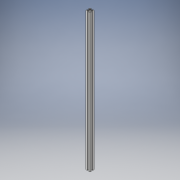
# Autodesk Inventor part: pro36in
Saved by Autodesk Inventor 2018 (Build 220112000, 112)
## iProperties
Created: 2017-09-02
Part Number: pro36in
Material: Generic
Document SubType Name: Modeling
Designer: snipe
Density: 1 g/cm^3
Appearance: Default
Author: snipe
Autodesk Inventor part; units mm, degrees
ref_plane "YZ Plane" through (0, 0, 0) normal (1, 0, 0) x (0, 1, 0)
ref_plane "XZ Plane" through (0, 0, 0) normal (0, 1, 0) x (-1, 0, 0)
ref_plane "XY Plane" through (0, 0, 0) normal (0, 0, 1) x (1, 0, 0)
sketch "Sketch1" plane through (0, 0, 0) normal (0, 1, 0) x (-1, 0, 0)
  line L0 (0, -14) -> (0, 14) projected
  line L1 (-14, 0) -> (14, 0) projected
  line L2 (14, 0) -> (-14, 0) projected
  line L3 (0, -14) -> (0, 14) projected
  line L4 (2.5943, 3.655) -> (-2.5943, 3.655)
  line L5 (-3.655, 2.5943) -> (-3.655, -2.5943)
  line L6 (-2.5943, -3.655) -> (2.5943, -3.655)
  line L7 (3.655, -2.5943) -> (3.655, 2.5943)
  line L8 (-3.655, 3.655) -> (3.655, -3.655) construction
  line L9 (10, 10) -> (10, 2.63)
  line L10 (10, 2.63) -> (8.5, 2.63)
  line L11 (10, 10) -> (2.63, 10)
  line L12 (2.63, 10) -> (2.63, 8.5)
  line L13 (-10, 10) -> (-2.63, 10)
  line L14 (-2.63, 10) -> (-2.63, 8.5)
  line L15 (-10, 8.5) -> (-10, 10)
  line L16 (-10, 10) -> (-8.5, 10)
  line L17 (-8.5, 2.63) -> (-10, 2.63)
  line L18 (-10, 2.63) -> (-10, 10)
  line L19 (-10, -10) -> (-8.5, -10)
  line L20 (-8.5, -2.63) -> (-10, -2.63)
  line L21 (-10, -2.63) -> (-10, -10)
  line L22 (-10, -10) -> (-2.63, -10)
  line L23 (-2.63, -10) -> (-2.63, -8.5)
  line L24 (-10, -8.5) -> (-10, -10)
  line L25 (10, -10) -> (8.5, -10)
  line L26 (8.5, -2.63) -> (10, -2.63)
  line L27 (10, -2.63) -> (10, -10)
  line L28 (10, -10) -> (2.63, -10)
  line L29 (2.63, -10) -> (2.63, -8.5)
  line L30 (10, -8.5) -> (10, -10)
  circle A0 centre (0, 0) radius 2.095
  line L31 (5.995, -10) -> (2.63, -10)
  line L32 (-2.63, -10) -> (-5.995, -10)
  line L33 (10, -10) -> (2.63, -10)
  line L34 (-2.63, -10) -> (-10, -10)
  line L35 (10, -5.995) -> (10, -2.63)
  line L36 (10, 2.63) -> (10, 5.995)
  line L37 (10, 10) -> (10, 2.63)
  line L38 (10, -2.63) -> (10, -10)
  line L39 (-5.995, 10) -> (-2.63, 10)
  line L40 (2.63, 10) -> (5.995, 10)
  line L41 (-10, 10) -> (-2.63, 10)
  line L42 (2.63, 10) -> (10, 10)
  line L43 (-10, 5.995) -> (-10, 2.63)
  line L44 (-10, -2.63) -> (-10, -5.995)
  line L45 (-10, -10) -> (-10, -2.63)
  line L46 (-10, 2.63) -> (-10, 10)
  line L47 (-2.63, -8.5) -> (-5.995, -8.5)
  line L48 (-8.5, -5.995) -> (-8.5, -2.63)
  line L49 (-8.5, -5.995) -> (-7.0557, -5.995)
  line L50 (-5.995, -8.5) -> (-5.995, -7.0557)
  line L51 (-5.995, 7.0557) -> (-5.995, 8.5)
  line L52 (2.63, 8.5) -> (5.995, 8.5)
  line L53 (8.5, 2.63) -> (8.5, 5.995)
  line L54 (8.5, 5.995) -> (7.0557, 5.995)
  line L55 (5.995, 8.5) -> (5.995, 7.0557)
  line L56 (2.63, -8.5) -> (5.995, -8.5)
  line L57 (9.5607, -8.5) -> (10, -8.5)
  line L58 (8.5, -10) -> (8.5, -9.5607)
  line L59 (8.5, -5.995) -> (8.5, -2.63)
  line L60 (7.0557, -5.995) -> (8.5, -5.995)
  line L61 (5.995, -7.0557) -> (5.995, -8.5)
  line L62 (3.655, 3.655) -> (-0.5303, -0.5303) construction
  line L63 (-1.4814, -1.4814) -> (-3.655, -3.655) construction
  line L64 (-8.5, 10) -> (-8.5, 9.5607)
  line L65 (-8.5, 5.995) -> (-8.5, 2.63)
  line L66 (-2.63, 8.5) -> (-5.995, 8.5)
  line L67 (-9.5607, 8.5) -> (-10, 8.5)
  line L68 (-7.0557, 5.995) -> (-8.5, 5.995)
  line L69 (-3.655, 2.5943) -> (-7.0557, 5.995)
  line L70 (-2.5943, 3.655) -> (-5.995, 7.0557)
  line L71 (5.995, 7.0557) -> (2.5943, 3.655)
  line L72 (7.0557, 5.995) -> (3.655, 2.5943)
  line L73 (7.0557, -5.995) -> (3.655, -2.5943)
  line L74 (5.995, -7.0557) -> (2.5943, -3.655)
  line L75 (-2.5943, -3.655) -> (-5.995, -7.0557)
  line L76 (-3.655, -2.5943) -> (-7.0557, -5.995)
  dimension "d26" = 4.19
  dimension "d0" = 20
  dimension "d1" = 20
  dimension "d2" = 7.31
  dimension "d3" = 7.31
  dimension "d4" = 20
  dimension "d5" = 11.99
  dimension "d6" = 11.99
  dimension "d11" = 7.37
  dimension "d12" = 1.5
  dimension "d13" = 7.37
  dimension "d14" = 1.5
  dimension "d15" = 7.37
  dimension "d16" = 1.5
  dimension "d17" = 7.37
  dimension "d18" = 1.5
  dimension "d19" = 7.37
  dimension "d20" = 7.37
  dimension "d21" = 1.5
  dimension "d22" = 1.5
  dimension "d23" = 7.37
  dimension "d24" = 7.37
  dimension "d25" = 1.5
  constraints: 146 end point, 42 parallel, 28 perpendicular, 13 horizontal, 2 midpoint, 2 point on line, 1 coincident, 3 other
  measures "d0" distance of L34.end L33.start
  measures "d1" distance of L33.start L9.start
  measures "d2" distance of L63.end L8.end
  measures "d3" distance of L8.start L63.end
  measures "d4" distance of L35.start L44.end
  measures "d5" distance of L44.end L43.start
  measures "d6" distance of L31.start L32.end
  measures "d11" distance of L9.end L9.start
  measures "d12" distance of L9.end L10.end
  measures "d13" distance of L9.start L11.end
  measures "d14" distance of L11.end L12.end
  measures "d15" distance of L14.end L15.start
  measures "d16" distance of L17.start L17.end
  measures "d17" distance of L16.end L17.start
  measures "d18" distance of L20.end L20.start
  measures "d19" distance of L20.start L19.end
  measures "d20" distance of L24.start L23.end
  measures "d21" distance of L23.end L22.end
  measures "d22" distance of L26.start L26.end
  measures "d23" distance of L25.end L26.start
  measures "d24" distance of L29.end L30.start
  measures "d25" distance of L28.end L29.end
extrude "Extrusion1" add sketch "Sketch1" along normal blind 660.4 contours L6 L75 L50 L47 L23 L22 L19 L21 L20 L48 L49 L76 L5 L1 A0 L0 | L0 A0 L1 L7 L73 L60 L59 L26 L27 L25 L28 L29 L56 L61 L74 L6 | L1 L5 L69 L68 L65 L17 L18 L15 L13 L14 L66 L51 L70 L4 L0 A0 | A0 L0 L4 L71 L55 L52 L12 L11 L9 L10 L53 L54 L72 L7 L1
fillet "Fillet1" radius 0.5 20 edges at (10, 330.2, 10) (2.63, 330.2, 10) (-2.63, 330.2, 10) (-2.63, 330.2, 8.5) (10, 330.2, 2.63) (8.5, 330.2, 2.63) (10, 330.2, -2.63) (8.5, 330.2, -2.63) (10, 330.2, -10) (2.63, 330.2, -8.5) (-2.63, 330.2, -10) (-2.63, 330.2, -8.5) (2.63, 330.2, -10) (-10, 330.2, -10) (-8.5, 330.2, -2.63) (-10, 330.2, -2.63) (-8.5, 330.2, 2.63) (-10, 330.2, 2.63) (-10, 330.2, 10) (2.63, 330.2, 8.5)
fillet "Fillet2" radius 0.75 24 edges at (-7.0557, 330.2, 5.995) (-3.655, 330.2, 2.5943) (-8.5, 330.2, -5.995) (-7.0557, 330.2, -5.995) (-5.995, 330.2, -8.5) (3.655, 330.2, -2.5943) (7.0557, 330.2, -5.995) (-2.5943, 330.2, 3.655) (-5.995, 330.2, 7.0557) (3.655, 330.2, 2.5943) (7.0557, 330.2, 5.995) (8.5, 330.2, 5.995) (8.5, 330.2, -5.995) (2.5943, 330.2, 3.655) (5.995, 330.2, 7.0557) (5.995, 330.2, 8.5) (-5.995, 330.2, 8.5) (-8.5, 330.2, 5.995) (2.5943, 330.2, -3.655) (5.995, 330.2, -7.0557) (5.995, 330.2, -8.5) (-5.995, 330.2, -7.0557) (-2.5943, 330.2, -3.655) (-3.655, 330.2, -2.5943)
body "Solid1"
